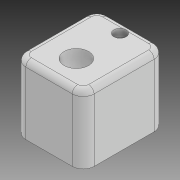
# Autodesk Inventor part: YIdler
Saved by Autodesk Inventor 2020 (Build 240168000, 168)
## iProperties
Created: 2020-10-29
Part Number: YIdler
Material: Generic
Document SubType Name: Modeling
Designer: DDeGo
Density: 1 g/cm^3
Appearance: Default
Author: DDeGo
Autodesk Inventor part; units mm, degrees
sketch "Sketch1" plane through (0, 0, 0) normal (1, 0, 0) x (0, 1, 0)
  line L0 (-12.5, 15) -> (12.5, 15)
  line L1 (12.5, 15) -> (12.5, -15)
  line L2 (12.5, -15) -> (-12.5, -15)
  line L3 (-12.5, -15) -> (-12.5, 15)
  line L4 (-12.5, 15) -> (12.5, -15) construction
  line L5 (12.5, 15) -> (-12.5, -15) construction
  point P0 (0, 0)
  dimension "d0" = 30
  dimension "d1" = 25
  constraints: 12 end point, 2 midpoint, 2 parallel, 1 horizontal, 1 perpendicular
  measures "d0" distance of L0.end L1.end
  measures "d1" distance of L1.end L2.end
extrude "Extrusion1" add sketch "Sketch1" along normal mid plane 25
sketch "Sketch5" plane through (-12.5, 12.5, 15) normal (0, 1, 0) x (1, 0, 0)
  line L0 (0, 30) -> (0, 0) projected
  line L1 (25, 0) -> (25, 30) projected
  circle A0 centre (12.5, 10) radius 2.65
  line L2 (12.5, 10) -> (12.5, 0) construction
  line L3 (0, 0) -> (25, 0) projected
  point P0 (12.5, 15)
  dimension "d22" = 5.3
  dimension "d25" = 10
  constraints: 2 end point, 1 centre point, 1 midpoint, 1 vertical, 1 other
  measures "d22" diameter of A0
  measures "d25" distance of L2.start L2.end
extrude "Extrusion5" cut sketch "Sketch5" against normal through all
ref_plane "Work Plane1" through (-12.5, 4.5, 15) normal (0, 1, 0) x (1, 0, 0)
sketch "Sketch2" plane through (-12.5, 4.5, 15) normal (0, 1, 0) x (1, 0, 0)
  circle A0 centre (12.5, 26) radius 9 construction
  circle A1 centre (12.5, 26) radius 1.75 construction
  line L0 (0, 30) -> (25, 30) construction
  line L1 (12.5, 30) -> (12.5, 26)
  circle A2 centre (12.5, 26) radius 10
  point P0 (12.5, 15)
  dimension "d5" = 4
  dimension "d6" = 3.5
  dimension "d7" = 18
  dimension "d8" = 1
  constraints: 3 centre point, 2 coincident, 2 end point, 1 midpoint, 1 vertical
  measures "d5" distance of L1.start L1.end
  measures "d6" diameter of A1
  measures "d7" diameter of A0
  measures "d8" radial gap between concentric circles of A0 A2
extrude "Extrusion2" cut sketch "Sketch2" against normal mid plane 11
sketch "Sketch3" plane through (-12.5, 4.5, 15) normal (0, 1, 0) x (1, 0, 0)
  arc A0 (3.3348, 30) -> (21.6652, 30) centre (12.5, 26) ccw projected
  circle A1 centre (12.5, 26) radius 2.25
  point P0 (12.5, 15)
  point P1 (20, 16)
  point P2 (0, 16)
  dimension "d11" = 4.5
  constraints: 1 centre point, 1 coincident
  measures "d11" diameter of A1
extrude "Extrusion3" cut sketch "Sketch3" along normal blind 10 and the other way blind 16
ref_plane "Work Plane2" through (-12.5, -2.5, 15) normal (0, 1, 0) x (1, 0, 0)
sketch "Sketch4" plane through (-12.5, -2.5, 15) normal (0, 1, 0) x (1, 0, 0)
  circle A0 centre (12.5, 26) radius 2.25 projected
  line L0 (12.5, 30.2147) -> (16.15, 28.1073) construction
  line L1 (16.15, 28.1073) -> (16.15, 23.8927)
  line L2 (16.15, 23.8927) -> (12.5, 21.7853)
  line L3 (12.5, 21.7853) -> (8.85, 23.8927)
  line L4 (8.85, 23.8927) -> (8.85, 28.1073)
  line L5 (8.85, 28.1073) -> (12.5, 30.2147) construction
  line L6 (8.85, 28.1073) -> (8.85, 36.3706)
  line L7 (8.85, 36.3706) -> (16.15, 36.3706)
  line L8 (16.15, 36.3706) -> (16.15, 28.1073)
  point P0 (12.5, 15)
  dimension "d46" = 7.3
  constraints: 18 end point, 2 perpendicular, 2 vertical, 1 coincident, 13 other
  measures "d46" distance between parallel lines of L1 L4
extrude "Extrusion4" cut sketch "Sketch4" against normal blind 3.5
fillet "Fillet1" radius 2 2 edges at (9.1652, 4.5, -15) (-9.1652, 4.5, -15)
fillet "Fillet1" radius 4 4 edges at (12.5, 0, -15) (-12.5, 0, -15) (-12.5, 0, 15) (12.5, 0, 15)
fillet "Fillet1" radius 2 4 edges at (12.5, 12.5, 0) (0, 12.5, 15) (-12.5, 12.5, 0) (0, 12.5, -15)
ref_plane "Work Plane3" through (-12.5, -7.5, -11) normal (0, -1, 0) x (1, 0, 0)
sketch "Sketch6" plane through (-12.5, -7.5, -11) normal (0, -1, 0) x (1, 0, 0)
  circle A0 centre (12.5, 16) radius 2.65 projected
  circle A1 centre (12.5, 16) radius 4.5
  point P0 (12.5, 11)
  dimension "d27" = 9
  constraints: 1 centre point, 1 coincident
  measures "d27" diameter of A1
extrude "Extrusion6" cut sketch "Sketch6" against normal through all contours A0 | A1
sketch "Sketch9" plane through (0, 0, 0) normal (1, 0, 0) x (0, 1, 0)
  line L0 (-17.5, -11) -> (17.5, -11) projected
  line L1 (-1, -8.75) -> (-1, -13.25) projected
  line L2 (10, -13.25) -> (10, -8.75) projected
  line L3 (10, -13.25) -> (10, -14.75)
  line L4 (10, -14.75) -> (9.5, -14.25)
  line L5 (9.5, -14.25) -> (9.5, -13.25)
  line L6 (9.5, -13.25) -> (10, -13.25)
  line L7 (-1, -13.25) -> (-0.5, -13.25)
  line L8 (-0.5, -13.25) -> (-0.5, -14.25)
  line L9 (-0.5, -14.25) -> (-1, -14.75)
  line L10 (-1, -14.75) -> (-1, -13.25)
  point P0 (0, 0)
  dimension "d38" = 0.5
  dimension "d39" = 1
  dimension "d40" = 45
  dimension "d41" = 0.5
  dimension "d42" = 1
  dimension "d43" = 45
  constraints: 16 end point, 2 parallel, 2 perpendicular, 1 point on line, 1 vertical
  measures "d38" distance of L5.end L2.start
  measures "d39" distance of L4.end L5.end
  measures "d40" angle of L3 L4
  measures "d41" distance of L1.end L7.end
  measures "d42" distance of L7.end L8.end
  measures "d43" angle of L10 L9
revolve "Revolution1" add sketch "Sketch9" angle 360 about axis through (0, 4.5, -11) along (0, 1, 0)
body "Solid1"
